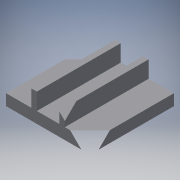
# Autodesk Inventor part: weight_holder_base
Saved by Autodesk Inventor 2016 (Build 200138000, 138)
## iProperties
Created: 2016-08-02
Part Number: weight_holder_base
Material: Generic
Document SubType Name: Sheet Metal
Designer: ajar021
Density: 1 g/cm^3
Appearance: Default
Sheet Metal Rule: Default
Author: ajar021
Autodesk Inventor part; units mm, degrees
ref_plane "YZ Plane" through (0, 0, 0) normal (1, 0, 0) x (0, 1, 0)
ref_plane "XZ Plane" through (0, 0, 0) normal (0, 1, 0) x (-1, 0, 0)
ref_plane "XY Plane" through (0, 0, 0) normal (0, 0, 1) x (1, 0, 0)
sketch "Sketch1" plane through (0, 0, 0) normal (0, 0, 1) x (1, 0, 0)
  line L0 (-7.5, 7.5) -> (7.5, 7.5)
  line L1 (7.5, 7.5) -> (7.5, -7.5)
  line L2 (7.5, -7.5) -> (-7.5, -7.5)
  line L3 (-7.5, -7.5) -> (-7.5, 7.5)
  line L4 (-7.5, 7.5) -> (7.5, -7.5) construction
  line L5 (7.5, 7.5) -> (-7.5, -7.5) construction
  point P0 (0, 0)
  dimension "d0" = 15
  dimension "d1" = 15
  constraints: 12 end point, 2 midpoint, 2 parallel, 1 horizontal, 1 perpendicular
  measures "d0" distance of L1.end L2.end
  measures "d1" distance of L0.end L1.end
extrude "Extrusion1" add sketch "Sketch1" along normal blind 2
sketch "Sketch2" plane through (0, 0, 2) normal (0, 0, 1) x (1, 0, 0)
  line L0 (-7.5, -7.5) -> (7.5, -7.5) projected
  line L1 (1.5, 7.5) -> (1.5, -7.5) construction
  line L2 (-1.5, -7.5) -> (-1.5, 7.5) construction
  line L3 (1.5, 7.5) -> (2, 7.5) construction
  line L4 (2, 7.5) -> (2, -7.5)
  line L5 (2, -7.5) -> (1.5, -7.5)
  line L6 (1.5, -7.5) -> (1.5, 7.5)
  line L7 (7.5, -7.5) -> (-7.5, -7.5) projected
  line L8 (-1.5, 7.5) -> (-2, 7.5)
  line L9 (-2, 7.5) -> (-2, -7.5)
  line L10 (-2, -7.5) -> (-1.5, -7.5)
  line L11 (-1.5, -7.5) -> (-1.5, 7.5)
  line L12 (7.5, 7.5) -> (-7.5, 7.5) projected
  line L13 (2, -7.5) -> (3, -7.5)
  line L14 (3, -7.5) -> (3, 7.5)
  line L15 (3, 7.5) -> (2, 7.5)
  line L16 (-2, 7.5) -> (-3, 7.5)
  line L17 (-3, 7.5) -> (-3, -7.5)
  line L18 (-2, -7.5) -> (-3, -7.5)
  point P0 (0, 0)
  dimension "d4" = 0.5
  dimension "d5" = 0.5
  dimension "d8" = 1
  dimension "d9" = 1
  constraints: 28 end point, 6 point on line, 4 parallel, 4 perpendicular, 2 collinear, 2 horizontal
  measures "d4" distance of L4.end L5.end
  measures "d5" distance of L10.end L9.end
  measures "d8" distance of L4.end L13.end
  measures "d9" distance of L8.end L16.end
extrude "Extrusion2" add sketch "Sketch2" along normal blind 3 contours L17 L12 L9 L0 | L4 L12 L14 L0
equation "\"d5\" = d4"
equation "\"d9\" = d8"
equation "\"BendRadius\" = Thickness"
equation "\"BendReliefWidth\" = Thickness"
equation "\"BendReliefDepth\" = 0.5 * Thickness"
equation "\"CornerReliefSize\" = 4 * Thickness"
equation "\"MinimumRemnant\" = 2 * Thickness"
equation "\"TransitionRadius\" = BendRadius"
equation "\"JacobiRadiusSize\" = Thickness"
equation "\"GapSize\" = Thickness"
equation "\"Thickness\" = 0.5"
body "Solid1"
